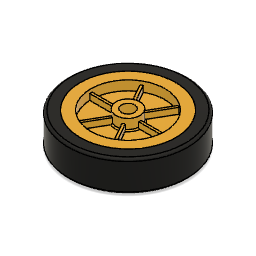
Roue (Autodesk Fusion 360 design; units mm, degrees)
Autodesk Fusion 360 part; units mm, degrees
sketch "Sketch1" plane through (0, 0, 0) normal (0, 1, 0) x (1, 0, 0)
  circle A0 centre (0, -55) radius 50
  circle A1 centre (0, -55) radius 40
  circle A2 centre (0, -55) radius 31
  circle A3 centre (0, -55) radius 5.5
  line L0 (0, -55) -> (31, -55)
  line L1 (0, -55) -> (15.5, -28.1532)
  line L2 (0, -55) -> (31, -55) construction
  line L3 (0, -55) -> (-15.5, -28.1532)
  line L4 (0, -55) -> (31, -55) construction
  line L5 (0, -55) -> (-31, -55)
  line L6 (0, -55) -> (15.5, -81.8468)
  line L7 (0, -55) -> (31, -55) construction
  line L8 (0, -55) -> (-15.5, -81.8468)
  line L9 (0, -55) -> (31, -55) construction
  line L10 (-0.866, -55.5) -> (-16.366, -28.6532)
  line L11 (-0.866, -55.5) -> (14.634, -82.3468)
  line L12 (0.866, -54.5) -> (-14.634, -27.6532)
  line L13 (0.866, -54.5) -> (16.366, -81.3468)
  line L14 (-0.866, -54.5) -> (14.634, -27.6532)
  line L15 (-0.866, -54.5) -> (-16.366, -81.3468)
  line L16 (0.866, -55.5) -> (16.366, -28.6532)
  line L17 (0.866, -55.5) -> (-14.634, -82.3468)
  line L18 (0, -56) -> (-31, -56)
  line L19 (0, -56) -> (31, -56)
  line L20 (0, -54) -> (-31, -54)
  line L21 (0, -54) -> (31, -54)
  circle A4 centre (0, -55) radius 10
  dimension "d1" = 100
  dimension "d2" = 80
  dimension "d3" = 62
  dimension "d4" = 11
  dimension "d5" = 31
  dimension "d6" = 60
  dimension "d7" = 120
  dimension "d8" = 31
  dimension "d9" = 60
  dimension "d10" = 120
  dimension "d11" = 1
  dimension "d12" = -1
  dimension "d13" = 1
  dimension "d14" = -1
  dimension "d15" = 1
  dimension "d16" = -1
  dimension "d17" = 20
  constraint concentric A0 A1
  constraint concentric A0 A2
  constraint concentric A2 A3
  constraint horizontal L0
  constraint coincident A0.centre A1.centre
  constraint horizontal L2
  constraint horizontal L4
  constraint horizontal L5
  constraint horizontal L7
  constraint horizontal L9
  constraint concentric A0 A4
  measures "d1" diameter of A0
  measures "d2" diameter of A1
  measures "d3" diameter of A2
  measures "d4" diameter of A3
  measures "d5" distance of A0.centre L1.end
  measures "d6" angle of L1 L2
  measures "d7" angle of L3 L4
  measures "d8" distance of A0.centre L5.end
  measures "d9" angle of L6 L7
  measures "d10" angle of L8 L9
  measures "d17" diameter of A4
extrude "Extrude1" add sketch "Sketch1" along normal mid plane 26 contours A0 makes body 1
extrude "Extrude2" add sketch "Sketch1" along normal mid plane 26 separate body contours A1 makes body 2
extrude "Extrude3" add sketch "Sketch1" along normal mid plane 10 contours A2 L16 L21 A4 | A2 L13 L19 A4 | A2 L12 L14 A4 | A2 L11 L17 A4 | A2 L10 L20 A4 | A2 L15 L18 A4 bodies 2
extrude "Extrude4" add sketch "Sketch1" along normal mid plane 20 contours A2 L0 L21 A4 | A2 L0 L19 A4 | A2 L1 L16 A4 | A2 L6 L13 A4 | A2 L1 L14 A4 | A2 L6 L11 A4 | A2 L3 L12 A4 | A2 L8 L17 A4 | A2 L3 L10 A4 | A2 L8 L15 A4 | A2 L5 L18 A4 | A2 L5 L20 A4 bodies 2
extrude "Extrude5" add sketch "Sketch1" along normal mid plane 28 contours A3 L0 L19 A4 | A3 L0 L21 A4 | A3 L16 L21 A4 | A3 L13 L19 A4 | A3 L1 L16 A4 | A3 L6 L13 A4 | A3 L1 L14 A4 | A3 L6 L11 A4 | A3 L12 L14 A4 | A3 L11 L17 A4 | A3 L3 L12 A4 | A3 L8 L17 A4 | A3 L3 L10 A4 | A3 L5 L20 A4 | A3 L5 L18 A4 | A3 L8 L15 A4 | A3 L10 L20 A4 | A3 L15 L18 A4 bodies 2
fillet "Fillet1" radius 2 2 edges at (-46.6164, 13, 73.0808) (-46.6164, -13, 36.9192) on bodies 1
fillet "Fillet2" radius 1 12 edges at (0, 5, 45) (-8.6603, 5, 50) (-8.6603, 5, 60) (0, 5, 65) (8.6603, 5, 50) (8.6603, 5, 60) (-8.6603, -5, 60) (-8.6603, -5, 50) (0, -5, 65) (8.6603, -5, 60) (0, -5, 45) (8.6603, -5, 50) on bodies 2
named bodies: "Grip", "Rim"
